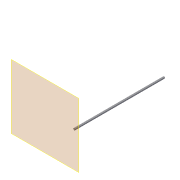
# Autodesk Inventor part: limit_swich_cover
Saved by Autodesk Inventor 2016 (Build 200138000, 138)
## iProperties
Created: 2016-08-18
Part Number: limit_swich_cover
Material: Generic
Document SubType Name: Modeling
Designer: admin
Density: 1 g/cm^3
Appearance: Default
Author: admin
Autodesk Inventor part; units mm, degrees
ref_plane "YZ Plane" through (0, 0, 0) normal (1, 0, 0) x (0, 1, 0)
ref_plane "XZ Plane" through (0, 0, 0) normal (0, 1, 0) x (-1, 0, 0)
ref_plane "XY Plane" through (0, 0, 0) normal (0, 0, 1) x (1, 0, 0)
ref_plane "Work Plane1" through (0, 0, 0) normal (0, 0, 1) x (1, 0, 0)
sketch "Sketch1" plane through (0, 0, 0) normal (0, 0, 1) x (1, 0, 0)
  arc A0 (180.3577, -7.1195) -> (184.0521, 3.2386) centre (67.5, 38.9711) ccw
  line L0 (177.8573, 4.3082) -> (182.3784, 3.5797) projected
  arc A1 (177.8573, 4.3082) -> (174.8842, -4.0274) centre (177.1414, -0.1344) ccw projected
  line L1 (178.8459, -6.3244) -> (174.8842, -4.0274) projected
  line L2 (184.0521, 3.2386) -> (182.3784, 3.5797)
  line L3 (178.8459, -6.3244) -> (180.3577, -7.1195)
  point P0 (0, 0)
  constraints: 4 end point, 2 point on circle, 1 centre point, 1 coincident
extrude "Extrusion1" add sketch "Sketch1" against normal blind 550
sketch "Sketch2" plane through (0, 0, 0) normal (0, 0, 1) x (1, 0, 0)
  arc A0 (180.3577, -7.1195) -> (184.0521, 3.2386) centre (67.5, 38.9711) ccw projected
  line L0 (182.3784, 3.5797) -> (184.0521, 3.2386) projected
  line L1 (177.8573, 4.3082) -> (182.3784, 3.5797) projected
  arc A1 (177.8573, 4.3082) -> (174.8842, -4.0274) centre (177.1414, -0.1344) ccw projected
  line L2 (178.8459, -6.3244) -> (174.8842, -4.0274) projected
  line L3 (180.3577, -7.1195) -> (178.8459, -6.3244) projected
  arc A2 (179.8349, -5.7419) -> (182.7755, 2.5028) centre (67.5, 38.9711) ccw
  line L4 (179.8349, -5.7419) -> (175.3858, -3.1623)
  arc A3 (177.6982, 3.321) -> (175.3858, -3.1623) centre (177.1414, -0.1344) ccw
  line L5 (177.6982, 3.321) -> (182.7755, 2.5028)
  point P0 (0, 0)
  dimension "d2" = 1
  constraints: 4 end point, 4 point on circle, 2 centre point, 3 other
  measures "d2" radial gap between concentric circles of A0 A2
extrude "Extrusion2" cut sketch "Sketch2" against normal blind 590 contours L4 A3 L5 A2
body "Solid1"
